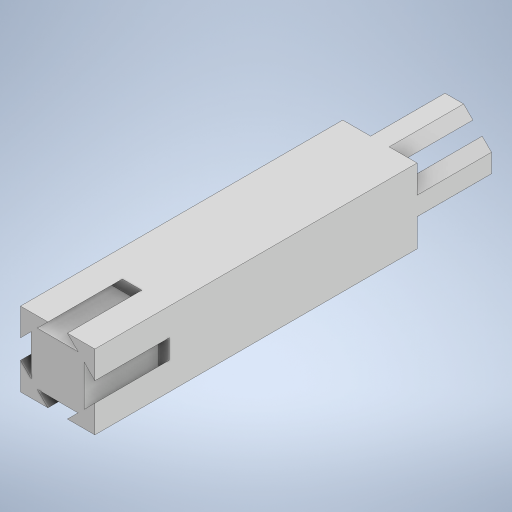
# Autodesk Inventor part: TestEbene2
Saved by Autodesk Inventor 2024 (Build 280153000, 153)
## iProperties
Created: 2025-01-15
Part Number: TestEbene2
Material: Generisch
Document SubType Name: Modeling
Designer: Carla
Density: 1 g/cm^3
Appearance: Vorgabe
Author: Carla
Autodesk Inventor part; units mm, degrees
ref_plane "YZ Plane" through (0, 0, 0) normal (1, 0, 0) x (0, 1, 0)
ref_plane "XZ Plane" through (0, 0, 0) normal (0, 1, 0) x (-1, 0, 0)
ref_plane "XY Plane" through (0, 0, 0) normal (0, 0, 1) x (1, 0, 0)
sketch "Skizze1" plane through (0, 0, 0) normal (0, 1, 0) x (-1, 0, 0)
  line L0 (15, 15) -> (-15, 15)
  line L1 (-15, 15) -> (-15, -15)
  line L2 (-15, -15) -> (15, -15)
  line L3 (15, -15) -> (15, 15)
  line L4 (15, 0) -> (11, 0) construction
  line L5 (11.25, 7.5042) -> (11.25, -7.4958)
  line L6 (15, 3.75) -> (15, -3.75)
  line L7 (11.25, 7.5042) -> (15, 3.75)
  line L8 (11.25, -7.4958) -> (15, -3.75)
  line L9 (-7.5042, 11.25) -> (-3.75, 15)
  line L10 (-7.5042, 11.25) -> (7.4958, 11.25)
  line L11 (7.4958, 11.25) -> (3.75, 15)
  line L12 (15, 15) -> (-15, 15)
  line L13 (-11.25, -7.5042) -> (-15, -3.75)
  line L14 (-11.25, -7.5042) -> (-11.25, 7.4958)
  line L15 (-11.25, 7.4958) -> (-15, 3.75)
  line L16 (-15, 15) -> (-15, -15)
  line L17 (7.5042, -11.25) -> (3.75, -15)
  line L18 (7.5042, -11.25) -> (-7.4958, -11.25)
  line L19 (-7.4958, -11.25) -> (-3.75, -15)
  line L20 (-15, -15) -> (15, -15)
  line L21 (15, -15) -> (-15, -15)
  line L22 (-15, -15) -> (-15, 15)
  line L23 (-15, 15) -> (15, 15)
  line L24 (15, 15) -> (15, -15)
  point P0 (0, 0)
  point P1 (0, 15)
  point P2 (-15, 0)
  point P3 (0, -15)
  point P4 (-3.75, -15)
  point P5 (3.75, -15)
  point P6 (-15, 3.75)
  point P7 (-15, -3.75)
  point P8 (3.75, 15)
  point P9 (-3.75, 15)
  dimension "d0" = 15
  dimension "d1" = 30
  dimension "d2" = 30
  dimension "d3" = 15
  dimension "d4" = 4
  dimension "d5" = 15
  dimension "d6" = 7.5
  dimension "d7" = 7.5
  dimension "d8" = 3.75
  dimension "d11" = 360
  constraints: 50 end point, 8 point on line, 4 parallel, 3 horizontal, 3 perpendicular, 1 midpoint, 1 vertical, 45 other
  measures "d0" distance from line of L3 point (0, 0)
  measures "d1" distance of L1.end L2.end
  measures "d2" distance of L2.end L0.start
  measures "d3" distance from line of point (0, 0) L2
  measures "d4" distance of L4.start L4.end
  measures "d5" distance of L5.start L5.end
  measures "d6" distance of L4.end L5.end
  measures "d7" distance of L6.start L6.end
  measures "d8" distance of L4.start L6.end
extrude "Extrusion1" add sketch "Skizze1" along normal blind 30 contours L11 L10 L9 L0 | L3 L8 L5 L7 | L15 L14 L13 L1 | L2 L19 L18 L17
extrude "Extrusion2" add sketch "Skizze1" against normal blind 70
sketch "Skizze4" plane through (0, -70, 0) normal (0, -1, 0) x (1, 0, 0)
  line L0 (-15.2121, -3.7121) -> (-10.7, -8.2243)
  line L1 (-10.7, -8.2243) -> (-10.7, 8.2243)
  line L2 (-10.7, 8.2243) -> (-15.2121, 3.7121)
  line L3 (-15, -3.9243) -> (-15, 3.9243)
  line L4 (3.7121, -15.2121) -> (8.2243, -10.7)
  line L5 (8.2243, -10.7) -> (-8.2243, -10.7)
  line L6 (-8.2243, -10.7) -> (-3.7121, -15.2121)
  line L7 (3.9243, -15) -> (-3.9243, -15)
  line L8 (15.2121, 3.7121) -> (10.7, 8.2243)
  line L9 (10.7, 8.2243) -> (10.7, -8.2243)
  line L10 (10.7, -8.2243) -> (15.2121, -3.7121)
  line L11 (15, 3.9243) -> (15, -3.9243)
  line L12 (-3.7121, 15.2121) -> (-8.2243, 10.7)
  line L13 (-8.2243, 10.7) -> (8.2243, 10.7)
  line L14 (8.2243, 10.7) -> (3.7121, 15.2121)
  line L15 (-3.9243, 15) -> (3.9243, 15)
  line L16 (-15, 15) -> (-3.75, 15) projected
  line L17 (-15, 15) -> (15, 15)
  line L18 (15, 15) -> (15, -15)
  line L19 (15, -15) -> (-15, -15)
  line L20 (-15, -15) -> (-15, 15)
  point P0 (0, 0)
  point P1 (0, 0)
  point P2 (-290.3305, 55.2757)
  point P3 (-298.179, 55.2757)
  point P4 (-3.9243, 15)
  dimension "d27" = 360
  constraints: 40 end point, 8 point on line, 2 parallel, 1 horizontal, 1 perpendicular, 41 other
extrude "Extrusion4" add sketch "Skizze4" along normal blind 30
sketch "Skizze5" plane through (0, -100, 0) normal (0, -1, 0) x (1, 0, 0)
  line L0 (18.5438, 0) -> (-21.4353, 0) construction
  line L1 (-11, 7.5) -> (-11, -7.5)
  line L2 (-11, 7.5) -> (-15, 3.5)
  line L3 (-11, -7.5) -> (-15, -3.5)
  line L4 (-15.2121, -3.7121) -> (-10.7, -8.2243)
  line L5 (-10.7, -8.2243) -> (-10.7, 8.2243)
  line L6 (-10.7, 8.2243) -> (-15.2121, 3.7121)
  line L7 (-15, -3.9243) -> (-15, 3.9243)
  line L8 (3.7121, -15.2121) -> (8.2243, -10.7)
  line L9 (8.2243, -10.7) -> (-8.2243, -10.7)
  line L10 (-8.2243, -10.7) -> (-3.7121, -15.2121)
  line L11 (3.9243, -15) -> (-3.9243, -15)
  line L12 (15.2121, 3.7121) -> (10.7, 8.2243)
  line L13 (10.7, 8.2243) -> (10.7, -8.2243)
  line L14 (10.7, -8.2243) -> (15.2121, -3.7121)
  line L15 (15, 3.9243) -> (15, -3.9243)
  line L16 (-3.7121, 15.2121) -> (-8.2243, 10.7)
  line L17 (-8.2243, 10.7) -> (8.2243, 10.7)
  line L18 (8.2243, 10.7) -> (3.7121, 15.2121)
  line L19 (-3.9243, 15) -> (3.9243, 15)
  line L20 (15, 15) -> (-15, 15) projected
  line L21 (3.9243, 15) -> (15, 15)
  line L22 (15, 15) -> (15, 3.9243)
  line L23 (15, -3.9243) -> (15, -15)
  line L24 (15, -15) -> (3.9243, -15)
  line L25 (-3.9243, -15) -> (-15, -15)
  line L26 (-15, -15) -> (-15, -3.9243)
  line L27 (-15, 3.9243) -> (-15, 15)
  line L28 (-15, 15) -> (-3.9243, 15)
  point P0 (0, 0)
  dimension "d34" = 15
  dimension "d38" = 0.3
  dimension "d39" = 360
  constraints: 56 end point, 12 point on line, 4 perpendicular, 2 horizontal, 1 collinear, 1 vertical, 43 other
  measures "d34" distance of L1.start L1.end
  measures "d38" distance between parallel lines of L3 L4
extrude "Extrusion5" add sketch "Skizze5" along normal blind 30 contours L27 L20 L16 L17 L18 L22 L12 L13 L14 L23 L24 L8 L9 L10 L25 L26 L4 L5 L6
equation "\"d0\" = 0.5 * d1"
equation "\"d3\" = 0.5 * d2"
equation "\"d6\" = 0.5 * d5"
equation "\"d8\" = 0.5 * d7"
